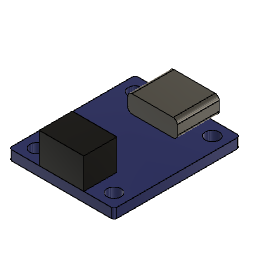
Adafruit Micro-Lipo Charger for LiPoly Batt with USB Type C Jack (Autodesk Fusion 360 design; units mm, degrees)
Autodesk Fusion 360 part; units mm, degrees
sketch "Sketch1" plane through (0, 0, 0) normal (0, 0, 1) x (1, 0, 0)
  line L0 (9.525, 11.43) -> (-9.525, 11.43)
  line L1 (-9.525, 11.43) -> (-9.525, -11.43)
  line L2 (-9.525, -11.43) -> (9.525, -11.43)
  line L3 (9.525, -11.43) -> (9.525, 11.43)
  line L4 (9.525, 11.43) -> (-9.525, -11.43) construction
  line L5 (-9.525, 11.43) -> (9.525, -11.43) construction
  dimension "d1" = 19.05
  dimension "d2" = 22.86
  constraint horizontal L0
  constraint perpendicular L0 L1
  constraint parallel L0 L2
  constraint parallel L1 L3
  constraint coincident L4 origin
  constraint coincident L5 origin
  measures "d1" distance of L0.start L0.end
  measures "d2" distance of L0.start L2.end
extrude "Extrude1" add sketch "Sketch1" along normal blind 1.75 makes body 1
sketch "Sketch2" plane through (0, 0, 1.75) normal (0, 0, 1) x (-1, 0, 0)
  line L0 (-9.525, 11.43) -> (-9.525, -11.43)
  line L1 (-9.525, -11.43) -> (9.525, -11.43)
  line L2 (9.525, -11.43) -> (9.525, 11.43)
  line L3 (9.525, 11.43) -> (-9.525, 11.43)
  line L4 (0, 11.43) -> (0, -11.43) construction
  line L5 (4.035, 11.43) -> (-4.035, 11.43)
  line L6 (-4.035, 11.43) -> (-4.035, 5.43)
  line L7 (-4.035, 5.43) -> (4.035, 5.43)
  line L8 (4.035, 5.43) -> (4.035, 11.43)
  dimension "d5" = 6
  dimension "d6" = 8.07
  constraint midpoint L3 L4.start
  constraint midpoint L1 L4.end
  constraint horizontal L5
  constraint vertical L6
  constraint horizontal L7
  constraint vertical L8
  constraint coincident L3 L5.start
  constraint midpoint L3 L5
  measures "d5" distance of L5.start L7.end
  measures "d6" distance of L6.end L7.end
extrude "Extrude2" add sketch "Sketch2" along normal blind 5.55 separate body contours L3 L5 L6 L7 L8 makes body 2
sketch "Sketch3" plane through (0, 0, 1.75) normal (0, 0, 1) x (-1, 0, 0)
  line L0 (-9.525, 11.43) -> (-9.525, -11.43)
  line L1 (-9.525, -11.43) -> (9.525, -11.43)
  line L2 (9.525, -11.43) -> (9.525, 11.43)
  line L3 (9.525, 11.43) -> (-9.525, 11.43)
  line L4 (4.485, -5.06) -> (-4.485, -5.06)
  line L5 (-4.485, -5.06) -> (-4.485, -12.66)
  line L6 (-4.485, -12.66) -> (4.485, -12.66)
  line L7 (4.485, -12.66) -> (4.485, -5.06)
  line L8 (0, -11.43) -> (0, 11.5) construction
  point P0 (0, -12.66)
  dimension "d9" = 7.6
  dimension "d10" = 8.97
  dimension "d11" = 1.23
  constraint horizontal L4
  constraint vertical L5
  constraint horizontal L6
  constraint vertical L7
  constraint midpoint L1 L8.start
  constraint perpendicular L3 L8
  constraint midpoint L6 P0
  constraint vertical L8.start P0
  measures "d9" distance of L4.start L6.end
  measures "d10" distance of L5.end L6.end
  measures "d11" distance of L1 L6
extrude "Extrude3" add sketch "Sketch3" along normal blind 3.2 separate body contours L1 L4 L5 L7 | L1 L5 L6 L7 makes body 3
fillet "Fillet1" radius 0.75 4 edges at (4.485, 8.86, 4.95) (4.485, 8.86, 1.75) (-4.485, 8.86, 4.95) (-4.485, 8.86, 1.75) on bodies 3
sketch "Sketch4" plane through (0, 0, 0) normal (0, 0, -1) x (1, 0, 0)
  line L0 (9.525, -11.43) -> (9.525, 11.43)
  line L1 (9.525, 11.43) -> (-9.525, 11.43)
  line L2 (-9.525, 11.43) -> (-9.525, -11.43)
  line L3 (-9.525, -11.43) -> (9.525, -11.43)
  circle A0 centre (-6.985, 8.89) radius 1.27
  line L4 (0, 0) -> (0, 11.43)
  line L5 (0, 0) -> (-9.525, 0)
  circle A1 centre (6.985, 8.89) radius 1.27
  circle A2 centre (6.985, -8.89) radius 1.27
  circle A3 centre (-6.985, -8.89) radius 1.27
  dimension "d15" = 2.54
  dimension "d21" = 13.97
  dimension "d22" = 17.78
  constraint coincident L4.start L5.start
  constraint midpoint L1 L4.end
  constraint midpoint L2 L5.end
  constraint symmetric A0 L4 A1
  constraint symmetric A0 L5 A3
  constraint symmetric L5 A1 A2
  measures "d15" diameter of A0
  measures "d21" distance of A2.centre A3.centre
  measures "d22" distance of A0.centre A3.centre
extrude "Extrude4" cut sketch "Sketch4" against normal up to surface (1.75 mm away) contours A0 | A1 | A2 | A3 bodies 1
fillet "Fillet2" radius 0.5 4 edges at (9.525, -11.43, 0.875) (-9.525, -11.43, 0.875) (-9.525, 11.43, 0.875) (9.525, 11.43, 0.875) on bodies 1
